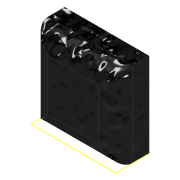
# Autodesk Inventor part: gom
Saved by Autodesk Inventor 2020.5 (Build 245400000, 400)
## iProperties
Created: 2022-11-30
Part Number: gom
Material: 一般
Document SubType Name: Modeling
Designer: Administrator
Density: 1 g/cm^3
Appearance: 黒
Author: Administrator
Autodesk Inventor part; units mm, degrees
ref_plane "YZ Plane" through (0, 0, 0) normal (1, 0, 0) x (0, 1, 0)
ref_plane "XZ Plane" through (0, 0, 0) normal (0, 1, 0) x (-1, 0, 0)
ref_plane "XY Plane" through (0, 0, 0) normal (0, 0, 1) x (1, 0, 0)
sketch "スケッチ2" plane through (0, 0, 0) normal (0, 0, 1) x (1, 0, 0)
  line L0 (25, -25) -> (25, 25) projected
  line L1 (25, 25) -> (-25, 25) projected
  line L2 (-25, 25) -> (-25, -25) projected
  line L3 (-25, -25) -> (25, -25) projected
  circle A0 centre (-20, 20) radius 2 projected
  circle A1 centre (20, 20) radius 2 projected
  circle A2 centre (20, -20) radius 2 projected
  ellipse E0 centre (0, 0) end of major axis (0, -14.1421) minor radius 10 projected
  circle A3 centre (-20, -20) radius 2 projected
  point P0 (0, 0)
  constraints: 1 other
extrude "押し出し1" add sketch "スケッチ2" along normal blind 20 contours L3 L2 L1 L0 | E0
sketch "スケッチ3" plane through (-25, -25, 0) normal (0, -1, 0) x (1, 0, 0)
  line L0 (0, 5) -> (50, 5) projected
  line L1 (0, 0) -> (50, 0) projected
  line L2 (50, 0) -> (50, 20) projected
  line L3 (0, 20) -> (50, 20) projected
  line L4 (0, 0) -> (0, 20) projected
  point P0 (25, 0)
fillet "フィレット1" radius 10 4 edges at (0, 25, 20) (25, 0, 20) (0, -25, 20) (-25, 0, 20)
